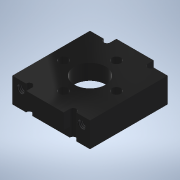
# Autodesk Inventor part: 頭_サーボホーンフレーム
Saved by Autodesk Inventor 2020 (Build 240168000, 168)
## iProperties
Created: 2016-05-04
Part Number: 頭_サーボホーンフレーム
Material: アセタール樹脂、黒
Document SubType Name: Modeling
Designer: hiroaki
Density: 1.425 g/cm^3
Appearance: 滑らか - 黒
Mass: 5.91414 g
Surface Area: 28.2108 cm^2
Volume: 4.15027 cm^3
Category: 頭
d0: 25.000 mm
d1: 1.050 mm
d2: 2.000 mm
d3: 6.500 mm
d4: 3.100 mm
d6: 3.000 mm
d14: 4.000 mm
d15: 0.00 deg
d17: 5.000 mm
d18: 5.000 mm
d21: 6.000 mm
d25: 8.800 mm
d27: 2.000 ul
d28: 360.00 deg
Author: hiroaki
Autodesk Inventor part; units mm, degrees
ref_plane "YZ Plane" through (0, 0, 0) normal (1, 0, 0) x (0, 1, 0)
ref_plane "XZ Plane" through (0, 0, 0) normal (0, 1, 0) x (-1, 0, 0)
ref_plane "XY Plane" through (0, 0, 0) normal (0, 0, 1) x (1, 0, 0)
sketch "スケッチ1" plane through (0, 0, 0) normal (0, 0, 1) x (1, 0, 0)
  line L0 (-12.5, -12.5) -> (12.5, -12.5) construction
  line L1 (12.5, -12.5) -> (12.5, 12.5) construction
  line L2 (12.5, 12.5) -> (-12.5, 12.5) construction
  line L3 (-12.5, 12.5) -> (-12.5, -12.5) construction
  line L4 (-12.5, -12.5) -> (12.5, 12.5) construction
  line L5 (12.5, -12.5) -> (-12.5, 12.5) construction
  line L6 (-8.1, 12.5) -> (-12.5, 12.5)
  line L7 (-12.5, 12.5) -> (-12.5, 8.1)
  line L8 (8.1, 12.5) -> (12.5, 12.5)
  line L9 (12.5, 12.5) -> (12.5, 8.1)
  line L10 (-12.5, -8.1) -> (-12.5, -12.5)
  line L11 (-12.5, -12.5) -> (-8.1, -12.5)
  line L12 (8.1, -12.5) -> (12.5, -12.5)
  line L13 (12.5, -12.5) -> (12.5, -8.1)
  line L14 (-6, 12.5) -> (-6, 14.5)
  line L15 (-6, 14.5) -> (6, 14.5)
  line L16 (6, 14.5) -> (6, 12.5)
  arc A0 (-8.1, 12.5) -> (-6, 12.5) centre (-7.05, 12.5) ccw
  arc A1 (6, 12.5) -> (8.1, 12.5) centre (7.05, 12.5) ccw
  line L17 (0, 12.5) -> (0, 0) construction
  line L18 (0, 0) -> (12.5, 0) construction
  line L19 (-12.5, 6) -> (-14.5, 6) construction
  line L20 (-14.5, 6) -> (-14.5, -6) construction
  line L21 (-14.5, -6) -> (-12.5, -6) construction
  arc A2 (-12.5, 6) -> (-12.5, 8.1) centre (-12.5, 7.05) ccw
  arc A3 (-12.5, -8.1) -> (-12.5, -6) centre (-12.5, -7.05) ccw construction
  line L22 (-6, -12.5) -> (-6, -14.5)
  line L23 (-6, -14.5) -> (6, -14.5)
  line L24 (6, -14.5) -> (6, -12.5)
  arc A4 (-6, -12.5) -> (-8.1, -12.5) centre (-7.05, -12.5) ccw
  arc A5 (8.1, -12.5) -> (6, -12.5) centre (7.05, -12.5) ccw
  line L25 (12.5, 6) -> (14.5, 6) construction
  line L26 (14.5, 6) -> (14.5, -6) construction
  line L27 (14.5, -6) -> (12.5, -6) construction
  arc A6 (12.5, 8.1) -> (12.5, 6) centre (12.5, 7.05) ccw construction
  arc A7 (12.5, -6) -> (12.5, -8.1) centre (12.5, -7.05) ccw construction
  line L28 (-9.05, 12.5) -> (-5.95, 12.5) construction
  line L29 (-5.95, 12.5) -> (-5.95, 9.5) construction
  line L30 (-5.95, 9.5) -> (-9.05, 9.5) construction
  line L31 (-9.05, 9.5) -> (-9.05, 12.5) construction
  line L32 (-12.5, 9.05) -> (-9.5, 9.05) construction
  line L33 (-9.5, 5.95) -> (-12.5, 5.95) construction
  line L34 (-12.5, 5.95) -> (-12.5, 9.05) construction
  line L35 (-7.5, 12.5) -> (-7.5, 9.5) construction
  line L36 (-9.5, 7.5) -> (-12.5, 7.5) construction
  line L37 (-12.5, -12.5) -> (-12.5, 12.5)
  line L38 (12.5, -12.5) -> (12.5, 12.5)
  dimension "d0" = 25
  dimension "d1" = 1.05
  dimension "d2" = 2
  dimension "d3" = 6.5
  dimension "d4" = 3.1
  dimension "d6" = 3
  dimension "d17" = 5
  dimension "d18" = 5
  dimension "d46" = 25
  constraints: 78 end point, 17 perpendicular, 16 point on circle, 8 centre point, 8 tangent, 7 equal radius, 7 horizontal, 7 midpoint, 6 collinear, 6 parallel, 6 symmetric about line, 4 horizontal alignment, 4 vertical, 4 vertical alignment, 6 other
  measures "d0" distance of L2.end L0.start
  measures "d1" radius of A0
  measures "d2" distance between parallel lines of L2 L15
  measures "d3" distance between parallel lines of L3 L14
  measures "d4" distance of L28.start L28.end
  measures "d6" distance between parallel lines of L6 L30
  measures "d17" distance between parallel lines of L2 L36
  measures "d18" distance between parallel lines of L7 L35
  measures "d46" distance of L1.end L2.end
extrude "押し出し1" add sketch "スケッチ1" along normal blind 4
mirror "ミラー1" about plane through (0, 0, 0) normal (0, 0, -1) of "押し出し1"
sketch "スケッチ2" plane through (-12.5, -12.5, 4) normal (0, -1, 0) x (1, 0, 0)
  line L0 (6.5, 0) -> (18.5, 0) construction
  line L1 (12.5, 0) -> (12.5, -5) construction
  line L2 (0, -8) -> (0, 0) construction
  line L3 (0, -2.5) -> (22.3, -2.5) construction
  point P0 (12.5, -4)
  point P1 (2.7, -2.5)
  point P2 (0.0223, -2.5)
  dimension "d52" = 2.7
  dimension "d53" = 2.5
  constraints: 4 end point, 2 horizontal alignment, 1 horizontal, 1 midpoint, 1 symmetric about line, 1 vertical, 2 other
  measures "d53" distance from line of point (0, 0) L3
hole "穴1" at (-9.8, -12.5, 1.5) at (9.8, -12.5, 1.5) direction (0, 1, 0) diameter 2.459 depth 8.8 thread size "M3x0.5" class "6H" standard "ISO Metric profile"
pattern_circular "円形状パターン1" count 2 over 360 about axis through (0, 0, -10) along (0, 0, 1) of "穴1"
sketch "スケッチ4" plane through (-8.1, -12.5, -4) normal (0, 0, -1) x (-1, 0, 0)
  circle A0 centre (-8.1, 4) radius 1.5
  line L0 (-8.1, 4) -> (-8.1, 12.5) construction
  circle A1 centre (0.4, 12.5) radius 1.5
  circle A2 centre (-8.1, 21) radius 1.5
  circle A3 centre (-16.6, 12.5) radius 1.5
  dimension "d35" = 3
  dimension "d36" = 8.5
  dimension "d39" = 360
  constraints: 4 centre point, 2 end point, 1 coincident, 1 vertical, 9 other
  measures "d35" diameter of A0
  measures "d36" distance of L0.start point (-8.1, 12.5)
extrude "押し出し3" cut sketch "スケッチ4" against normal through all
sketch "スケッチ5" plane through (-8.1, -12.5, -4) normal (0, 0, -1) x (-1, 0, 0)
  circle A0 centre (-8.1, 12.5) radius 5.05
  dimension "d43" = 10.1
  constraints: 1 centre point, 1 coincident
  measures "d43" diameter of A0
extrude "押し出し4" cut sketch "スケッチ5" against normal blind 2
sketch "スケッチ6" plane through (0, 0, 4) normal (0, 0, 1) x (1, 0, 0)
  circle A0 centre (8.5, 0) radius 1.5 construction
  circle A1 centre (0, 8.5) radius 1.5 construction
  circle A2 centre (-8.5, 0) radius 1.5 construction
  circle A3 centre (0, -8.5) radius 1.5 construction
  line L0 (0, -8.5) -> (0, 8.5) construction
  line L1 (8.5, 0) -> (-8.5, 0) construction
  circle A4 centre (0, 0) radius 5.05
  dimension "d47" = 10.1
  constraints: 4 end point, 1 centre point, 1 coincident, 1 horizontal, 1 vertical
  measures "d47" diameter of A4
extrude "押し出し5" cut sketch "スケッチ6" against normal up to surface (8 mm away)
sketch "スケッチ8" plane through (6, 14.5, -4) normal (0, 0, -1) x (-1, 0, 0)
  line L0 (0, -29) -> (0, -27) projected
  line L1 (12, -29) -> (0, -29) projected
  line L2 (12, -27) -> (12, -29) projected
  line L3 (0, 0) -> (12, 0) projected
  line L4 (0, -2) -> (0, 0) projected
  line L5 (12, 0) -> (12, -2) projected
  line L6 (0, -27) -> (12, -27)
  line L7 (0, -2) -> (12, -2)
  circle A0 centre (6, -14.5) radius 10.51
  dimension "d54" = 21.02
  constraints: 4 end point, 1 centre point, 1 coincident, 1 horizontal, 1 perpendicular
  measures "d54" diameter of A0
extrude "押し出し6" cut sketch "スケッチ8" against normal blind 3
equation "\"d18\" = d17"
